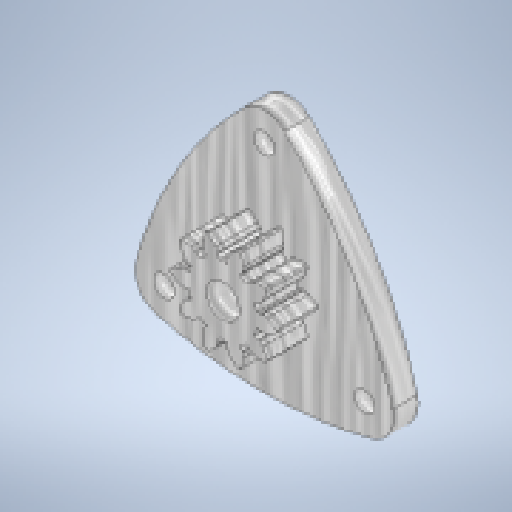
# Autodesk Inventor part: m1z10t8
Saved by Autodesk Inventor 2023 (Build 270158030, 158C)
## iProperties
Created: 2022-06-26
Part Number: m1z10t8
Material: アルミニウム 7075
Document SubType Name: Modeling
Designer: muzho
Density: 2.81 g/cm^3
Appearance: サテン - ブラシ仕上げ 重厚
Mass: 6.76867 g
Surface Area: 21.4239 cm^2
Volume: 2.40878 cm^3
Author: muzho
Autodesk Inventor part; units mm, degrees
ref_plane "YZ Plane" through (0, 0, 0) normal (1, 0, 0) x (0, 1, 0)
ref_plane "XZ Plane" through (0, 0, 0) normal (0, 1, 0) x (-1, 0, 0)
ref_plane "XY Plane" through (0, 0, 0) normal (0, 0, 1) x (1, 0, 0)
sketch "スケッチ1" plane through (0, 0, 0) normal (0, 0, 1) x (1, 0, 0)
  arc A0 (13.8322, -3.0794) -> (9.583, -10.4393) centre (12.9904, -7.5) ccw construction
  arc A1 (9.201, -13.3942) -> (9.583, -10.4393) centre (8.0686, -11.7457) ccw construction
  arc A2 (-9.201, -13.3942) -> (9.201, -13.3942) centre (0, 0) ccw construction
  arc A3 (-9.583, -10.4393) -> (-9.201, -13.3942) centre (-8.0686, -11.7457) ccw construction
  arc A4 (-9.583, -10.4393) -> (-13.8322, -3.0794) centre (-12.9904, -7.5) ccw construction
  arc A5 (-16.2002, -1.2712) -> (-13.8322, -3.0794) centre (-14.2063, -1.1147) ccw construction
  arc A6 (-6.9992, 14.6654) -> (-16.2002, -1.2712) centre (0, 0) ccw construction
  arc A7 (-4.2492, 13.5188) -> (-6.9992, 14.6654) centre (-6.1378, 12.8604) ccw construction
  arc A8 (-4.2492, 13.5188) -> (4.2492, 13.5187) centre (0, 15) ccw construction
  arc A9 (6.9992, 14.6654) -> (4.2492, 13.5187) centre (6.1378, 12.8604) ccw construction
  arc A10 (16.2002, -1.2712) -> (6.9992, 14.6654) centre (0, 0) ccw construction
  arc A11 (13.8322, -3.0794) -> (16.2002, -1.2712) centre (14.2063, -1.1147) ccw construction
  circle A12 centre (12.9904, -7.5) radius 1.5 construction
  circle A13 centre (-12.9904, -7.5) radius 1.5 construction
  circle A14 centre (0, 0) radius 18.25 construction
  circle A15 centre (0, 14) radius 3.5
  circle A16 centre (-12.1244, -7) radius 3.5
  circle A17 centre (12.1244, -7) radius 3.5
  arc A18 (-2.4699, 16.4798) -> (-15.5069, -6.1009) centre (32.815, -18.9458) ccw
  arc A19 (-13.0369, -10.3789) -> (13.0369, -10.3789) centre (0, 37.8915) ccw
  arc A20 (15.5069, -6.1009) -> (2.4699, 16.4798) centre (-32.815, -18.9458) ccw
  circle A21 centre (0, 0) radius 2
  circle A22 centre (0, 14) radius 1.25
  circle A23 centre (-12.1244, -7) radius 1.25
  circle A24 centre (12.1244, -7) radius 1.25
  point P0 (15.5069, -6.1009)
  point P1 (2.4699, 16.4798)
  point P2 (-13.0369, -10.3789)
  dimension "d21" = 7
  dimension "d3" = 360
  dimension "d5" = 50
  dimension "d8" = 360
  dimension "d10" = 4
  dimension "d15" = 2.5
  dimension "d18" = 360
  dimension "d20" = 14
  constraints: 30 point on circle, 23 centre point, 2 coincident, 1 vertical alignment, 79 other
  measures "d5" radius of A18
  measures "d10" diameter of A21
  measures "d15" diameter of A22
  measures "d20" distance of point (0, 0) point (0, 14)
extrude "押し出し1" add sketch "スケッチ1" along normal blind 2.5
sketch "スケッチ2" plane through (0, 0, 2.5) normal (0, 0, 1) x (1, 0, 0)
  arc A0 (0.5556, 4.8181) -> (0.5131, 4.6704) centre (1.1772, 4.5593) ccw
  arc A1 (0.8331, 5.2927) -> (0.5556, 4.8181) centre (2.3167, 4.1066) ccw
  arc A2 (1.8568, 6.1598) -> (0.8331, 5.2927) centre (3.5506, 3.1222) ccw
  arc A3 (-2.3825, 4.2245) -> (-2.3301, 4.08) centre (-1.7275, 4.3805) ccw
  arc A4 (-2.437, 4.7715) -> (-2.3825, 4.2245) centre (-0.5396, 4.6841) ccw
  arc A5 (-2.1184, 6.0748) -> (-2.437, 4.7715) centre (1.0373, 4.6129) ccw
  arc A6 (-4.4106, 2.0173) -> (-4.2832, 1.9312) centre (-3.9723, 2.5285) ccw
  arc A7 (-4.7762, 2.4278) -> (-4.4106, 2.0173) centre (-3.1898, 3.4723) ccw
  arc A8 (-5.2845, 3.6694) -> (-4.7762, 2.4278) centre (-1.8722, 4.3416) ccw
  arc A9 (-4.754, -0.9605) -> (-4.6003, -0.9553) centre (-4.6999, -0.2893) ccw
  arc A10 (-5.2911, -0.8432) -> (-4.754, -0.9605) centre (-4.6215, 0.9343) ccw
  arc A11 (-6.4321, -0.1375) -> (-5.2911, -0.8432) centre (-4.0666, 2.412) ccw
  arc A12 (-3.2815, -3.5714) -> (-3.1603, -3.4768) centre (-3.6323, -2.9966) ccw
  arc A13 (-3.7849, -3.7922) -> (-3.2815, -3.5714) centre (-4.2881, -1.9606) ccw
  arc A14 (-5.1228, -3.892) -> (-3.7849, -3.7922) centre (-4.7077, -0.439) ccw
  arc A15 (-0.5556, -4.8181) -> (-0.5131, -4.6704) centre (-1.1772, -4.5593) ccw
  arc A16 (-0.8331, -5.2927) -> (-0.5556, -4.8181) centre (-2.3167, -4.1066) ccw
  arc A17 (-1.8568, -6.1598) -> (-0.8331, -5.2927) centre (-3.5506, -3.1222) ccw
  arc A18 (2.3825, -4.2245) -> (2.3301, -4.08) centre (1.7275, -4.3805) ccw
  arc A19 (2.437, -4.7715) -> (2.3825, -4.2245) centre (0.5396, -4.6841) ccw
  arc A20 (2.1184, -6.0748) -> (2.437, -4.7715) centre (-1.0373, -4.6129) ccw
  arc A21 (4.4106, -2.0173) -> (4.2832, -1.9312) centre (3.9723, -2.5285) ccw
  arc A22 (4.7762, -2.4278) -> (4.4106, -2.0173) centre (3.1898, -3.4723) ccw
  arc A23 (5.2845, -3.6694) -> (4.7762, -2.4278) centre (1.8722, -4.3416) ccw
  arc A24 (4.754, 0.9605) -> (4.6003, 0.9553) centre (4.6999, 0.2893) ccw
  arc A25 (5.2911, 0.8432) -> (4.754, 0.9605) centre (4.6215, -0.9343) ccw
  arc A26 (6.4321, 0.1375) -> (5.2911, 0.8432) centre (4.0666, -2.412) ccw
  arc A27 (3.2815, 3.5714) -> (3.1603, 3.4768) centre (3.6323, 2.9966) ccw
  arc A28 (3.7849, 3.7922) -> (3.2815, 3.5714) centre (4.2881, 1.9606) ccw
  arc A29 (5.1228, 3.892) -> (3.7849, 3.7922) centre (4.7077, 0.439) ccw
  arc A30 (-0.5131, 4.6704) -> (-0.5556, 4.8181) centre (-1.1772, 4.5593) ccw
  arc A31 (-0.5556, 4.8181) -> (-0.8331, 5.2927) centre (-2.3167, 4.1066) ccw
  arc A32 (-0.8331, 5.2927) -> (-1.8568, 6.1598) centre (-3.5506, 3.1222) ccw
  arc A33 (-3.1603, 3.4768) -> (-3.2815, 3.5714) centre (-3.6323, 2.9966) ccw
  arc A34 (-3.2815, 3.5714) -> (-3.7849, 3.7922) centre (-4.2881, 1.9606) ccw
  arc A35 (-3.7849, 3.7922) -> (-5.1228, 3.892) centre (-4.7077, 0.439) ccw
  arc A36 (-4.6003, 0.9553) -> (-4.754, 0.9605) centre (-4.6999, 0.2893) ccw
  arc A37 (-4.754, 0.9605) -> (-5.2911, 0.8432) centre (-4.6215, -0.9343) ccw
  arc A38 (-5.2911, 0.8432) -> (-6.4321, 0.1375) centre (-4.0666, -2.412) ccw
  arc A39 (-4.2832, -1.9312) -> (-4.4106, -2.0173) centre (-3.9723, -2.5285) ccw
  arc A40 (-4.4106, -2.0173) -> (-4.7762, -2.4278) centre (-3.1898, -3.4723) ccw
  arc A41 (-4.7762, -2.4278) -> (-5.2845, -3.6694) centre (-1.8722, -4.3416) ccw
  arc A42 (-2.3301, -4.08) -> (-2.3825, -4.2245) centre (-1.7275, -4.3805) ccw
  arc A43 (-2.3825, -4.2245) -> (-2.437, -4.7715) centre (-0.5396, -4.6841) ccw
  arc A44 (-2.437, -4.7715) -> (-2.1184, -6.0748) centre (1.0373, -4.6129) ccw
  arc A45 (0.5131, -4.6704) -> (0.5556, -4.8181) centre (1.1772, -4.5593) ccw
  arc A46 (0.5556, -4.8181) -> (0.8331, -5.2927) centre (2.3167, -4.1066) ccw
  arc A47 (0.8331, -5.2927) -> (1.8568, -6.1598) centre (3.5506, -3.1222) ccw
  arc A48 (3.1603, -3.4768) -> (3.2815, -3.5714) centre (3.6323, -2.9966) ccw
  arc A49 (3.2815, -3.5714) -> (3.7849, -3.7922) centre (4.2881, -1.9606) ccw
  arc A50 (3.7849, -3.7922) -> (5.1228, -3.892) centre (4.7077, -0.439) ccw
  arc A51 (4.6003, -0.9553) -> (4.754, -0.9605) centre (4.6999, -0.2893) ccw
  arc A52 (4.754, -0.9605) -> (5.2911, -0.8432) centre (4.6215, 0.9343) ccw
  arc A53 (5.2911, -0.8432) -> (6.4321, -0.1375) centre (4.0666, 2.412) ccw
  arc A54 (4.2832, 1.9312) -> (4.4106, 2.0173) centre (3.9723, 2.5285) ccw
  arc A55 (4.4106, 2.0173) -> (4.7762, 2.4278) centre (3.1898, 3.4723) ccw
  arc A56 (4.7762, 2.4278) -> (5.2845, 3.6694) centre (1.8722, 4.3416) ccw
  arc A57 (2.3301, 4.08) -> (2.3825, 4.2245) centre (1.7275, 4.3805) ccw
  arc A58 (2.3825, 4.2245) -> (2.437, 4.7715) centre (0.5396, 4.6841) ccw
  arc A59 (2.437, 4.7715) -> (2.1184, 6.0748) centre (-1.0373, 4.6129) ccw
  arc A60 (0.4586, 4.1749) -> (-0.4586, 4.1749) centre (0, 0) ccw
  arc A61 (-2.0829, 3.6471) -> (-2.825, 3.108) centre (0, 0) ccw
  arc A62 (-3.8288, 1.7263) -> (-4.1123, 0.8539) centre (0, 0) ccw
  arc A63 (-4.1123, -0.8539) -> (-3.8288, -1.7263) centre (0, 0) ccw
  arc A64 (-2.825, -3.108) -> (-2.0829, -3.6471) centre (0, 0) ccw
  arc A65 (-0.4586, -4.1749) -> (0.4586, -4.1749) centre (0, 0) ccw
  arc A66 (2.0829, -3.6471) -> (2.825, -3.108) centre (0, 0) ccw
  arc A67 (3.8288, -1.7263) -> (4.1123, -0.8539) centre (0, 0) ccw
  arc A68 (4.1123, 0.8539) -> (3.8288, 1.7263) centre (0, 0) ccw
  arc A69 (2.825, 3.108) -> (2.0829, 3.6471) centre (0, 0) ccw
  arc A70 (-1.8568, 6.1598) -> (-2.1184, 6.0748) centre (0, 0) ccw
  arc A71 (-5.1228, 3.892) -> (-5.2845, 3.6694) centre (0, 0) ccw
  arc A72 (-6.4321, 0.1375) -> (-6.4321, -0.1375) centre (0, 0) ccw
  arc A73 (-5.2845, -3.6694) -> (-5.1228, -3.892) centre (0, 0) ccw
  arc A74 (-2.1184, -6.0748) -> (-1.8568, -6.1598) centre (0, 0) ccw
  arc A75 (1.8568, -6.1598) -> (2.1184, -6.0748) centre (0, 0) ccw
  arc A76 (5.1228, -3.892) -> (5.2845, -3.6694) centre (0, 0) ccw
  arc A77 (6.4321, -0.1375) -> (6.4321, 0.1375) centre (0, 0) ccw
  arc A78 (5.2845, 3.6694) -> (5.1228, 3.892) centre (0, 0) ccw
  arc A79 (2.1184, 6.0748) -> (1.8568, 6.1598) centre (0, 0) ccw
  line L0 (0.4586, 4.1749) -> (0.5131, 4.6704)
  line L1 (-2.0829, 3.6471) -> (-2.3301, 4.08)
  line L2 (-3.8288, 1.7263) -> (-4.2832, 1.9312)
  line L3 (-4.1123, -0.8539) -> (-4.6003, -0.9553)
  line L4 (-2.825, -3.108) -> (-3.1603, -3.4768)
  line L5 (-0.4586, -4.1749) -> (-0.5131, -4.6704)
  line L6 (2.0829, -3.6471) -> (2.3301, -4.08)
  line L7 (3.8288, -1.7263) -> (4.2832, -1.9312)
  line L8 (4.1123, 0.8539) -> (4.6003, 0.9553)
  line L9 (2.825, 3.108) -> (3.1603, 3.4768)
  line L10 (-0.4586, 4.1749) -> (-0.5131, 4.6704)
  line L11 (-2.825, 3.108) -> (-3.1603, 3.4768)
  line L12 (-4.1123, 0.8539) -> (-4.6003, 0.9553)
  line L13 (-3.8288, -1.7263) -> (-4.2832, -1.9312)
  line L14 (-2.0829, -3.6471) -> (-2.3301, -4.08)
  line L15 (0.4586, -4.1749) -> (0.5131, -4.6704)
  line L16 (2.825, -3.108) -> (3.1603, -3.4768)
  line L17 (4.1123, -0.8539) -> (4.6003, -0.9553)
  line L18 (3.8288, 1.7263) -> (4.2832, 1.9312)
  line L19 (2.0829, 3.6471) -> (2.3301, 4.08)
  circle A80 centre (0, 0) radius 2 projected
  constraints: 160 point on circle, 80 centre point, 40 end point
extrude "押し出し2" add sketch "スケッチ2" along normal blind 5
